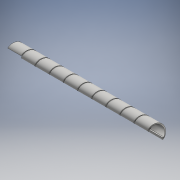
# Autodesk Inventor part: magicAngle5
Saved by Autodesk Inventor 2016 (Build 200138000, 138)
## iProperties
Created: 2025-04-04
Part Number: magicAngle5
Material: Generic
Document SubType Name: Modeling
Designer: iraklisrigakis
Density: 1 g/cm^3
Appearance: Default
Author: iraklisrigakis
Autodesk Inventor part; units mm, degrees
ref_plane "YZ Plane" through (0, 0, 0) normal (1, 0, 0) x (0, 1, 0)
ref_plane "XZ Plane" through (0, 0, 0) normal (0, 1, 0) x (-1, 0, 0)
ref_plane "XY Plane" through (0, 0, 0) normal (0, 0, 1) x (1, 0, 0)
sketch "Sketch1" plane through (0, 0, 0) normal (0, 0, 1) x (1, 0, 0)
  line L0 (0, 0.5) -> (-9.0815, 0.5)
  line L1 (0, -5.5) -> (21.5, -5.5)
  line L2 (21.5, -5.5) -> (21.5, -7.3)
  line L3 (21.5, -7.3) -> (0, -7.3)
  line L4 (0, -7.3) -> (0, -5.5)
  line L5 (0, -5.5) -> (0, 0.5)
  point P0 (0, 0)
  dimension "d2" = 1.8
  dimension "d14" = 6
  constraints: 12 end point, 2 horizontal, 2 parallel, 1 perpendicular, 1 vertical
  measures "d2" distance of L1.end L2.end
  measures "d14" distance of L1.start L5.end
coil "Coil1" sketch "Sketch1" operation add axis through (0, 0.5, 0) along (-1, 0, 0) pitch 22.7 turns 10 hand left
body "Solid1"
